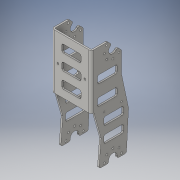
# Autodesk Inventor part: Tungkak
Saved by Autodesk Inventor 2016 (Build 200138000, 138)
## iProperties
Created: 2017-02-15
Part Number: Tungkak
Material: Generic
Document SubType Name: Modeling
Designer: Ghana
Density: 1 g/cm^3
Appearance: Default
Author: Ghana
Autodesk Inventor part; units mm, degrees
note: some values were not read from the file. Chosen so that the rebuilt part matches the saved one: bend side of "Bend Part3".
ref_plane "YZ Plane" through (0, 0, 0) normal (1, 0, 0) x (0, 1, 0)
ref_plane "XZ Plane" through (0, 0, 0) normal (0, 1, 0) x (-1, 0, 0)
ref_plane "XY Plane" through (0, 0, 0) normal (0, 0, 1) x (1, 0, 0)
sketch "Sketch5" plane through (0, 0, 0) normal (0, 0, 1) x (1, 0, 0)
  line L0 (0, 0) -> (2, 0)
  line L1 (2, 0) -> (2, 70)
  line L2 (2, 70) -> (0, 70)
  line L3 (0, 70) -> (0, 0)
  line L4 (2, 70) -> (18.6716, 70)
  line L5 (2, 0) -> (2, 70)
  line L6 (20.0858, 69.4142) -> (22.9467, 66.5533)
  line L7 (37, 51.6716) -> (37, 26.405)
  arc A0 (22.2396, 63.0178) -> (30.0178, 55.2396) centre (26.1287, 59.1287) ccw
  line L8 (22.2396, 63.0178) -> (22.9467, 63.7249)
  line L9 (30.0178, 55.2396) -> (30.7249, 55.9467)
  line L10 (33.5533, 55.9467) -> (36.4142, 53.0858)
  line L11 (10.6287, -65) -> (18.6287, -65)
  line L12 (31.6287, -63) -> (31.6287, -62)
  line L13 (20.6287, -62) -> (20.6287, -63)
  arc A1 (31.6287, -62) -> (20.6287, -62) centre (26.1287, -62) ccw
  line L14 (33.6287, -65) -> (41.6287, -65)
  arc A2 (8.6287, -63) -> (10.6287, -65) centre (10.6287, -63) ccw
  arc A3 (41.6287, -65) -> (43.6287, -63) centre (41.6287, -63) ccw
  arc A4 (22.9467, 63.7249) -> (22.9467, 66.5533) centre (21.5325, 65.1391) ccw
  arc A5 (33.5533, 55.9467) -> (30.7249, 55.9467) centre (32.1391, 54.5325) ccw
  arc A6 (20.0858, 69.4142) -> (18.6716, 70) centre (18.6716, 68) ccw
  arc A7 (37, 51.6716) -> (36.4142, 53.0858) centre (35, 51.6716) ccw
  arc A8 (18.6287, -65) -> (20.6287, -63) centre (18.6287, -63) ccw
  arc A9 (31.6287, -63) -> (33.6287, -65) centre (33.6287, -63) ccw
  line L15 (37, 26.405) -> (46.0883, -16.2505)
  line L16 (46.0883, -16.2505) -> (43.6287, -63)
  line L17 (11.0883, -32.3022) -> (8.6287, -63)
  line L18 (2, 0) -> (11.0883, -32.3022)
  circle A10 centre (18.3505, 66.9069) radius 1.25
  circle A11 centre (15.1287, 59.1287) radius 1.25
  circle A12 centre (18.3505, 51.3505) radius 1.25
  circle A13 centre (26.1287, 48.1287) radius 1.25
  circle A14 centre (33.9069, 51.3505) radius 1.25
  circle A15 centre (37.1287, -62) radius 1.25
  circle A16 centre (33.9069, -54.2218) radius 1.25
  circle A17 centre (26.1287, -51) radius 1.25
  circle A18 centre (18.3505, -54.2218) radius 1.25
  circle A19 centre (15.1287, -62) radius 1.25
  line L19 (8.5442, 39.2835) -> (29.5442, 39.2835)
  line L20 (31.5442, 37.2835) -> (31.5442, 31.2835)
  line L21 (29.5442, 29.2835) -> (8.5442, 29.2835)
  line L22 (6.5442, 31.2835) -> (6.5442, 37.2835)
  line L23 (8.5442, 14.2835) -> (29.5442, 14.2835)
  line L24 (31.5442, 12.2835) -> (31.5442, 6.2835)
  line L25 (29.5442, 4.2835) -> (8.5442, 4.2835)
  line L26 (6.5442, 6.2835) -> (6.5442, 12.2835)
  circle A20 centre (14.6287, -5.1373) radius 1
  circle A21 centre (37.1287, -5.1373) radius 1
  line L27 (16.6287, -10.7165) -> (37.6287, -10.7165)
  line L28 (39.6287, -12.7165) -> (39.6287, -18.7165)
  line L29 (37.6287, -20.7165) -> (16.6287, -20.7165)
  line L30 (14.6287, -18.7165) -> (14.6287, -12.7165)
  line L31 (16.6287, -30.7165) -> (37.6287, -30.7165)
  line L32 (39.6287, -32.7165) -> (39.6287, -38.7165)
  line L33 (37.6287, -40.7165) -> (16.6287, -40.7165)
  line L34 (14.6287, -38.7165) -> (14.6287, -32.7165)
  arc A22 (8.5442, 39.2835) -> (6.5442, 37.2835) centre (8.5442, 37.2835) ccw
  arc A23 (31.5442, 37.2835) -> (29.5442, 39.2835) centre (29.5442, 37.2835) ccw
  arc A24 (29.5442, 29.2835) -> (31.5442, 31.2835) centre (29.5442, 31.2835) ccw
  arc A25 (6.5442, 31.2835) -> (8.5442, 29.2835) centre (8.5442, 31.2835) ccw
  arc A26 (8.5442, 14.2835) -> (6.5442, 12.2835) centre (8.5442, 12.2835) ccw
  arc A27 (31.5442, 12.2835) -> (29.5442, 14.2835) centre (29.5442, 12.2835) ccw
  arc A28 (29.5442, 4.2835) -> (31.5442, 6.2835) centre (29.5442, 6.2835) ccw
  arc A29 (6.5442, 6.2835) -> (8.5442, 4.2835) centre (8.5442, 6.2835) ccw
  arc A30 (16.6287, -10.7165) -> (14.6287, -12.7165) centre (16.6287, -12.7165) ccw
  arc A31 (39.6287, -12.7165) -> (37.6287, -10.7165) centre (37.6287, -12.7165) ccw
  arc A32 (37.6287, -20.7165) -> (39.6287, -18.7165) centre (37.6287, -18.7165) ccw
  arc A33 (14.6287, -18.7165) -> (16.6287, -20.7165) centre (16.6287, -18.7165) ccw
  arc A34 (39.6287, -32.7165) -> (37.6287, -30.7165) centre (37.6287, -32.7165) ccw
  arc A35 (37.6287, -40.7165) -> (39.6287, -38.7165) centre (37.6287, -38.7165) ccw
  arc A36 (14.6287, -38.7165) -> (16.6287, -40.7165) centre (16.6287, -38.7165) ccw
  arc A37 (16.6287, -30.7165) -> (14.6287, -32.7165) centre (16.6287, -32.7165) ccw
  line L35 (-44.454, 0) -> (-46.454, 0)
  line L36 (-46.454, 0) -> (-46.454, 70)
  line L37 (-46.454, 70) -> (-44.454, 70)
  line L38 (-44.454, 70) -> (-44.454, 0)
  line L39 (-46.454, 70) -> (-63.1256, 70)
  line L40 (-46.454, 0) -> (-46.454, 70)
  line L41 (-64.5398, 69.4142) -> (-67.4007, 66.5533)
  line L42 (-81.454, 51.6716) -> (-81.454, 26.405)
  arc A38 (-74.4718, 55.2396) -> (-66.6936, 63.0178) centre (-70.5827, 59.1287) ccw
  line L43 (-66.6936, 63.0178) -> (-67.4007, 63.7249)
  line L44 (-74.4718, 55.2396) -> (-75.1789, 55.9467)
  line L45 (-78.0073, 55.9467) -> (-80.8682, 53.0858)
  line L46 (-55.0827, -65) -> (-63.0827, -65)
  line L47 (-76.0827, -63) -> (-76.0827, -62)
  line L48 (-65.0827, -62) -> (-65.0827, -63)
  arc A39 (-65.0827, -62) -> (-76.0827, -62) centre (-70.5827, -62) ccw
  line L49 (-78.0827, -65) -> (-86.0827, -65)
  arc A40 (-55.0827, -65) -> (-53.0827, -63) centre (-55.0827, -63) ccw
  arc A41 (-88.0827, -63) -> (-86.0827, -65) centre (-86.0827, -63) ccw
  arc A42 (-67.4007, 66.5533) -> (-67.4007, 63.7249) centre (-65.9865, 65.1391) ccw
  arc A43 (-75.1789, 55.9467) -> (-78.0073, 55.9467) centre (-76.5931, 54.5325) ccw
  arc A44 (-63.1256, 70) -> (-64.5398, 69.4142) centre (-63.1256, 68) ccw
  arc A45 (-80.8682, 53.0858) -> (-81.454, 51.6716) centre (-79.454, 51.6716) ccw
  arc A46 (-65.0827, -63) -> (-63.0827, -65) centre (-63.0827, -63) ccw
  arc A47 (-78.0827, -65) -> (-76.0827, -63) centre (-78.0827, -63) ccw
  line L50 (-81.454, 26.405) -> (-90.5423, -16.2505)
  line L51 (-90.5423, -16.2505) -> (-88.0827, -63)
  line L52 (-55.5423, -32.3022) -> (-53.0827, -63)
  line L53 (-46.454, 0) -> (-55.5423, -32.3022)
  circle A48 centre (-62.8045, 66.9069) radius 1.25
  circle A49 centre (-59.5827, 59.1287) radius 1.25
  circle A50 centre (-62.8045, 51.3505) radius 1.25
  circle A51 centre (-70.5827, 48.1287) radius 1.25
  circle A52 centre (-78.3609, 51.3505) radius 1.25
  circle A53 centre (-81.5827, -62) radius 1.25
  circle A54 centre (-78.3609, -54.2218) radius 1.25
  circle A55 centre (-70.5827, -51) radius 1.25
  circle A56 centre (-62.8045, -54.2218) radius 1.25
  circle A57 centre (-59.5827, -62) radius 1.25
  line L54 (-52.9982, 39.2835) -> (-73.9982, 39.2835)
  line L55 (-75.9982, 37.2835) -> (-75.9982, 31.2835)
  line L56 (-73.9982, 29.2835) -> (-52.9982, 29.2835)
  line L57 (-50.9982, 31.2835) -> (-50.9982, 37.2835)
  line L58 (-52.9982, 14.2835) -> (-73.9982, 14.2835)
  line L59 (-75.9982, 12.2835) -> (-75.9982, 6.2835)
  line L60 (-73.9982, 4.2835) -> (-52.9982, 4.2835)
  line L61 (-50.9982, 6.2835) -> (-50.9982, 12.2835)
  circle A58 centre (-59.0827, -5.1373) radius 1
  circle A59 centre (-81.5827, -5.1373) radius 1
  line L62 (-61.0827, -10.7165) -> (-82.0827, -10.7165)
  line L63 (-84.0827, -12.7165) -> (-84.0827, -18.7165)
  line L64 (-82.0827, -20.7165) -> (-61.0827, -20.7165)
  line L65 (-59.0827, -18.7165) -> (-59.0827, -12.7165)
  line L66 (-61.0827, -30.7165) -> (-82.0827, -30.7165)
  line L67 (-84.0827, -32.7165) -> (-84.0827, -38.7165)
  line L68 (-82.0827, -40.7165) -> (-61.0827, -40.7165)
  line L69 (-59.0827, -38.7165) -> (-59.0827, -32.7165)
  arc A60 (-50.9982, 37.2835) -> (-52.9982, 39.2835) centre (-52.9982, 37.2835) ccw
  arc A61 (-73.9982, 39.2835) -> (-75.9982, 37.2835) centre (-73.9982, 37.2835) ccw
  arc A62 (-75.9982, 31.2835) -> (-73.9982, 29.2835) centre (-73.9982, 31.2835) ccw
  arc A63 (-52.9982, 29.2835) -> (-50.9982, 31.2835) centre (-52.9982, 31.2835) ccw
  arc A64 (-50.9982, 12.2835) -> (-52.9982, 14.2835) centre (-52.9982, 12.2835) ccw
  arc A65 (-73.9982, 14.2835) -> (-75.9982, 12.2835) centre (-73.9982, 12.2835) ccw
  arc A66 (-75.9982, 6.2835) -> (-73.9982, 4.2835) centre (-73.9982, 6.2835) ccw
  arc A67 (-52.9982, 4.2835) -> (-50.9982, 6.2835) centre (-52.9982, 6.2835) ccw
  arc A68 (-59.0827, -12.7165) -> (-61.0827, -10.7165) centre (-61.0827, -12.7165) ccw
  arc A69 (-82.0827, -10.7165) -> (-84.0827, -12.7165) centre (-82.0827, -12.7165) ccw
  arc A70 (-84.0827, -18.7165) -> (-82.0827, -20.7165) centre (-82.0827, -18.7165) ccw
  arc A71 (-61.0827, -20.7165) -> (-59.0827, -18.7165) centre (-61.0827, -18.7165) ccw
  arc A72 (-82.0827, -30.7165) -> (-84.0827, -32.7165) centre (-82.0827, -32.7165) ccw
  arc A73 (-84.0827, -38.7165) -> (-82.0827, -40.7165) centre (-82.0827, -38.7165) ccw
  arc A74 (-61.0827, -40.7165) -> (-59.0827, -38.7165) centre (-61.0827, -38.7165) ccw
  arc A75 (-59.0827, -32.7165) -> (-61.0827, -30.7165) centre (-61.0827, -32.7165) ccw
  line L70 (0, 0) -> (-44.454, 0)
  line L71 (-44.454, 0) -> (-44.454, 70)
  line L72 (-44.454, 70) -> (0, 70)
  line L73 (0, 70) -> (0, 0)
  line L74 (-32.454, 60) -> (-12, 60)
  line L75 (-10, 58) -> (-10, 52)
  line L76 (-12, 50) -> (-32.454, 50)
  line L77 (-34.454, 52) -> (-34.454, 58)
  line L78 (-32.454, 40) -> (-12, 40)
  line L79 (-10, 38) -> (-10, 32)
  line L80 (-12, 30) -> (-32.454, 30)
  line L81 (-34.454, 32) -> (-34.454, 38)
  line L82 (-32.454, 20) -> (-12, 20)
  line L83 (-10, 18) -> (-10, 12)
  line L84 (-12, 10) -> (-32.454, 10)
  line L85 (-34.454, 12) -> (-34.454, 18)
  circle A76 centre (-39.454, 35) radius 1.25
  circle A77 centre (-5, 35) radius 1.25
  arc A78 (-32.454, 40) -> (-34.454, 38) centre (-32.454, 38) ccw
  arc A79 (-10, 38) -> (-12, 40) centre (-12, 38) ccw
  arc A80 (-12, 30) -> (-10, 32) centre (-12, 32) ccw
  arc A81 (-34.454, 32) -> (-32.454, 30) centre (-32.454, 32) ccw
  arc A82 (-32.454, 60) -> (-34.454, 58) centre (-32.454, 58) ccw
  arc A83 (-10, 58) -> (-12, 60) centre (-12, 58) ccw
  arc A84 (-12, 50) -> (-10, 52) centre (-12, 52) ccw
  arc A85 (-34.454, 52) -> (-32.454, 50) centre (-32.454, 52) ccw
  arc A86 (-32.454, 20) -> (-34.454, 18) centre (-32.454, 18) ccw
  arc A87 (-10, 18) -> (-12, 20) centre (-12, 18) ccw
  arc A88 (-12, 10) -> (-10, 12) centre (-12, 12) ccw
  arc A89 (-34.454, 12) -> (-32.454, 10) centre (-32.454, 12) ccw
  point P0 (32.1391, 57.3609)
  point P1 (31.5442, 29.2835)
  point P2 (31.5442, 39.2835)
  point P3 (6.5442, 14.2835)
  point P4 (31.5442, 4.2835)
  point P5 (31.5442, 14.2835)
  point P6 (39.6287, -20.7165)
  point P7 (39.6287, -10.7165)
  point P8 (39.6287, -40.7165)
  point P9 (39.6287, -30.7165)
  point P10 (-76.5931, 57.3609)
  point P11 (-75.9982, 29.2835)
  point P12 (-75.9982, 39.2835)
  point P13 (-50.9982, 14.2835)
  point P14 (-75.9982, 4.2835)
  point P15 (-75.9982, 14.2835)
  point P16 (-84.0827, -20.7165)
  point P17 (-84.0827, -10.7165)
  point P18 (-84.0827, -40.7165)
  point P19 (-84.0827, -30.7165)
  point P20 (-10, 50)
  point P21 (-10, 60)
  point P22 (-10, 30)
  point P23 (-10, 40)
  point P24 (-10, 10)
  point P25 (-10, 20)
  dimension "d110" = 2
  dimension "d121" = 2
  dimension "d122" = 2
  dimension "d128" = 2.5
  dimension "d131" = 180
  dimension "d137" = 180
  dimension "d140" = 10
  dimension "d141" = 10
  dimension "d144" = 10
  dimension "d145" = 15
  dimension "d146" = 15
  dimension "d147" = 10
  dimension "d148" = 10
  dimension "d154" = 10
  dimension "d155" = 10
  dimension "d156" = 10
  dimension "d157" = 10
  dimension "d158" = 10
  dimension "d161" = 2.5
  dimension "d162" = 2
  constraints: 172 end point, 130 point on circle, 90 centre point, 72 tangent, 58 point on line, 32 equal radius, 20 parallel, 14 perpendicular, 12 horizontal, 18 other
  measures "d110" distance of L2.end L1.end
  measures "d121" radius of A2
  measures "d122" radius of A6
  measures "d128" diameter of A10
  measures "d140" distance of point (31.544, 39.284) point (31.544, 29.284)
  measures "d141" distance of point (31.544, 14.284) point (31.544, 4.284)
  measures "d144" distance of point (39.629, -10.716) point (39.629, -20.716)
  measures "d145" distance between parallel lines of L23 L21
  measures "d146" distance between parallel lines of L27 L25
  measures "d147" distance of point (39.629, -30.716) point (39.629, -40.716)
  measures "d148" distance between parallel lines of L31 L29
  measures "d154" distance of point (-10, 60) point (-10, 50)
  measures "d155" distance of point (-10, 40) point (-10, 30)
  measures "d156" distance of point (-10, 20) point (-10, 10)
  measures "d157" distance between parallel lines of L70 L84
  measures "d158" distance between parallel lines of L82 L80
  measures "d161" diameter of A76
  measures "d162" radius of A78
extrude "Extrusion2" add sketch "Sketch5" along normal blind 2
sketch "Sketch6" plane through (0, 0, 0) normal (0, 0, -1) x (-1, 0, 0)
  line L0 (0, 0) -> (0, 70)
  line L1 (-18.6716, 70) -> (63.1256, 70) projected
  constraints: 2 end point, 1 point on line, 1 vertical
bend part "Bend Part3" radius 1.2732 angle 90 line through (0, 0, 0) along (0, 1, 0) centre toward (0, 0, -1) moving side (1, 0, 0) both sides no
sketch "Sketch7" plane through (0, 0, 0) normal (0, 0, -1) x (-1, 0, 0)
  line L0 (0, 0) -> (0, 70) projected
  line L1 (46.454, 0) -> (0, 0) projected
  line L2 (55.5423, -32.3022) -> (46.454, 0) projected
  line L3 (53.0827, -63) -> (55.5423, -32.3022) projected
  arc A0 (53.0827, -63) -> (55.0827, -65) centre (55.0827, -63) ccw projected
  line L4 (63.0827, -65) -> (55.0827, -65) projected
  arc A1 (63.0827, -65) -> (65.0827, -63) centre (63.0827, -63) ccw projected
  line L5 (65.0827, -62) -> (65.0827, -63) projected
  arc A2 (76.0827, -62) -> (65.0827, -62) centre (70.5827, -62) ccw projected
  line L6 (76.0827, -63) -> (76.0827, -62) projected
  arc A3 (76.0827, -63) -> (78.0827, -65) centre (78.0827, -63) ccw projected
  line L7 (86.0827, -65) -> (78.0827, -65) projected
  arc A4 (86.0827, -65) -> (88.0827, -63) centre (86.0827, -63) ccw projected
  line L8 (90.5423, -16.2505) -> (88.0827, -63) projected
  line L9 (81.454, 26.405) -> (90.5423, -16.2505) projected
  line L10 (81.454, 51.6716) -> (81.454, 26.405) projected
  arc A5 (81.454, 51.6716) -> (80.8682, 53.0858) centre (79.454, 51.6716) ccw projected
  line L11 (78.0073, 55.9467) -> (80.8682, 53.0858) projected
  arc A6 (78.0073, 55.9467) -> (75.1789, 55.9467) centre (76.5931, 54.5325) ccw projected
  line L12 (74.4718, 55.2396) -> (75.1789, 55.9467) projected
  arc A7 (66.6936, 63.0178) -> (74.4718, 55.2396) centre (70.5827, 59.1287) ccw projected
  line L13 (67.4007, 63.7249) -> (66.6936, 63.0178) projected
  arc A8 (67.4007, 63.7249) -> (67.4007, 66.5533) centre (65.9865, 65.1391) ccw projected
  line L14 (64.5398, 69.4142) -> (67.4007, 66.5533) projected
  arc A9 (64.5398, 69.4142) -> (63.1256, 70) centre (63.1256, 68) ccw projected
  line L15 (0, 70) -> (63.1256, 70) projected
  arc A10 (61.0827, -10.7165) -> (59.0827, -12.7165) centre (61.0827, -12.7165) ccw projected
  line L16 (61.0827, -10.7165) -> (82.0827, -10.7165) projected
  arc A11 (84.0827, -12.7165) -> (82.0827, -10.7165) centre (82.0827, -12.7165) ccw projected
  line L17 (84.0827, -12.7165) -> (84.0827, -18.7165) projected
  arc A12 (82.0827, -20.7165) -> (84.0827, -18.7165) centre (82.0827, -18.7165) ccw projected
  line L18 (82.0827, -20.7165) -> (61.0827, -20.7165) projected
  arc A13 (59.0827, -18.7165) -> (61.0827, -20.7165) centre (61.0827, -18.7165) ccw projected
  line L19 (59.0827, -18.7165) -> (59.0827, -12.7165) projected
  arc A14 (52.9982, 14.2835) -> (50.9982, 12.2835) centre (52.9982, 12.2835) ccw projected
  line L20 (52.9982, 14.2835) -> (73.9982, 14.2835) projected
  arc A15 (75.9982, 12.2835) -> (73.9982, 14.2835) centre (73.9982, 12.2835) ccw projected
  line L21 (75.9982, 12.2835) -> (75.9982, 6.2835) projected
  arc A16 (73.9982, 4.2835) -> (75.9982, 6.2835) centre (73.9982, 6.2835) ccw projected
  line L22 (73.9982, 4.2835) -> (52.9982, 4.2835) projected
  arc A17 (50.9982, 6.2835) -> (52.9982, 4.2835) centre (52.9982, 6.2835) ccw projected
  line L23 (50.9982, 6.2835) -> (50.9982, 12.2835) projected
  arc A18 (82.0827, -40.7165) -> (84.0827, -38.7165) centre (82.0827, -38.7165) ccw projected
  line L24 (82.0827, -40.7165) -> (61.0827, -40.7165) projected
  arc A19 (59.0827, -38.7165) -> (61.0827, -40.7165) centre (61.0827, -38.7165) ccw projected
  line L25 (59.0827, -38.7165) -> (59.0827, -32.7165) projected
  arc A20 (61.0827, -30.7165) -> (59.0827, -32.7165) centre (61.0827, -32.7165) ccw projected
  line L26 (61.0827, -30.7165) -> (82.0827, -30.7165) projected
  arc A21 (84.0827, -32.7165) -> (82.0827, -30.7165) centre (82.0827, -32.7165) ccw projected
  line L27 (84.0827, -32.7165) -> (84.0827, -38.7165) projected
  arc A22 (50.9982, 31.2835) -> (52.9982, 29.2835) centre (52.9982, 31.2835) ccw projected
  line L28 (50.9982, 31.2835) -> (50.9982, 37.2835) projected
  arc A23 (52.9982, 39.2835) -> (50.9982, 37.2835) centre (52.9982, 37.2835) ccw projected
  line L29 (52.9982, 39.2835) -> (73.9982, 39.2835) projected
  arc A24 (75.9982, 37.2835) -> (73.9982, 39.2835) centre (73.9982, 37.2835) ccw projected
  line L30 (75.9982, 37.2835) -> (75.9982, 31.2835) projected
  arc A25 (73.9982, 29.2835) -> (75.9982, 31.2835) centre (73.9982, 31.2835) ccw projected
  line L31 (73.9982, 29.2835) -> (52.9982, 29.2835) projected
  circle A26 centre (70.5827, 48.1287) radius 1.25 projected
  circle A27 centre (78.3609, 51.3505) radius 1.25 projected
  circle A28 centre (62.8045, 51.3505) radius 1.25 projected
  circle A29 centre (62.8045, 66.9069) radius 1.25 projected
  circle A30 centre (59.5827, 59.1287) radius 1.25 projected
  circle A31 centre (81.5827, -62) radius 1.25 projected
  circle A32 centre (59.5827, -62) radius 1.25 projected
  circle A33 centre (62.8045, -54.2218) radius 1.25 projected
  circle A34 centre (78.3609, -54.2218) radius 1.25 projected
  circle A35 centre (70.5827, -51) radius 1.25 projected
  circle A36 centre (81.5827, -5.1373) radius 1 projected
  circle A37 centre (59.0827, -5.1373) radius 1 projected
  arc A38 (12, 20) -> (10, 18) centre (12, 18) ccw projected
  line L32 (12, 20) -> (32.454, 20) projected
  arc A39 (34.454, 18) -> (32.454, 20) centre (32.454, 18) ccw projected
  line L33 (34.454, 18) -> (34.454, 12) projected
  arc A40 (32.454, 10) -> (34.454, 12) centre (32.454, 12) ccw projected
  line L34 (32.454, 10) -> (12, 10) projected
  arc A41 (10, 12) -> (12, 10) centre (12, 12) ccw projected
  line L35 (10, 12) -> (10, 18) projected
  arc A42 (12, 60) -> (10, 58) centre (12, 58) ccw projected
  line L36 (12, 60) -> (32.454, 60) projected
  arc A43 (34.454, 58) -> (32.454, 60) centre (32.454, 58) ccw projected
  line L37 (34.454, 58) -> (34.454, 52) projected
  arc A44 (32.454, 50) -> (34.454, 52) centre (32.454, 52) ccw projected
  line L38 (32.454, 50) -> (12, 50) projected
  arc A45 (10, 52) -> (12, 50) centre (12, 52) ccw projected
  line L39 (10, 52) -> (10, 58) projected
  arc A46 (12, 40) -> (10, 38) centre (12, 38) ccw projected
  line L40 (12, 40) -> (32.454, 40) projected
  arc A47 (34.454, 38) -> (32.454, 40) centre (32.454, 38) ccw projected
  line L41 (34.454, 38) -> (34.454, 32) projected
  arc A48 (32.454, 30) -> (34.454, 32) centre (32.454, 32) ccw projected
  line L42 (32.454, 30) -> (12, 30) projected
  arc A49 (10, 32) -> (12, 30) centre (12, 32) ccw projected
  line L43 (10, 32) -> (10, 38) projected
  circle A50 centre (5, 35) radius 1.25 projected
  circle A51 centre (39.454, 35) radius 1.25 projected
  line L44 (55.5423, -32.3022) -> (46.454, 0) projected
  line L45 (0, 70) -> (63.1256, 70) projected
  line L46 (46.454, 0) -> (44.454, 0)
  line L47 (44.454, 0) -> (44.454, 70)
  line L48 (44.454, 70) -> (46.454, 70)
  line L49 (46.454, 70) -> (46.454, 0)
  dimension "d167" = 2
  constraints: 8 end point, 2 parallel, 1 horizontal, 1 perpendicular, 1 point on line
  measures "d167" distance of L47.end L48.end
bend part "Bend Part4" radius 1.2732 angle 90 line through (-44.454, 0, 0) along (0, 1, 0) centre toward (0, 0, -1) moving side (-1, 0, 0) both sides no
body "Solid2"
